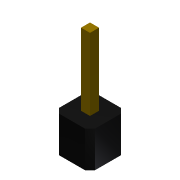
# Autodesk Inventor part: Header1x1
Saved by Autodesk Inventor 2013 (Build 170138000, 138)
## iProperties
Created: 2013-01-19
Part Number: Header1x1
Material: Generic
Document SubType Name: Modeling
Designer: davidgitz
Density: 1 g/cm^3
Author: davidgitz
Autodesk Inventor part; units mm, degrees
ref_plane "YZ Plane" through (0, 0, 0) normal (1, 0, 0) x (0, 1, 0)
ref_plane "XZ Plane" through (0, 0, 0) normal (0, 1, 0) x (-1, 0, 0)
ref_plane "XY Plane" through (0, 0, 0) normal (0, 0, 1) x (1, 0, 0)
sketch "Sketch1" plane through (0, 0, 0) normal (0, 1, 0) x (-1, 0, 0)
  line L0 (0.9108, 1.27) -> (-0.9108, 1.27)
  line L1 (-0.9108, 1.27) -> (-1.27, 0.9108)
  line L2 (-1.27, 0.9108) -> (-1.27, -0.9108)
  line L3 (0.9108, -1.27) -> (1.27, -0.9108)
  line L4 (1.27, -0.9108) -> (1.27, 0.9108)
  line L5 (0.9108, 1.27) -> (1.27, 0.9108)
  line L6 (-1.27, -0.9108) -> (-0.9108, -1.27)
  line L7 (-0.9108, -1.27) -> (0.9108, -1.27)
  line L8 (-1.27, 0) -> (1.27, 0) construction
  point P0 (0, 0)
  point P1 (0, 0)
  dimension "d1" = 2.54
  dimension "d3" = 0.508
  dimension "d4" = 135
  constraints: 18 end point, 10 perpendicular, 3 midpoint, 1 coincident, 1 vertical
  measures "d1" distance between parallel lines of L4 L2
  measures "d3" distance of L0.end L1.end
  measures "d4" angle of L0 L1
extrude "Extrusion1" add sketch "Sketch1" along normal blind 2.54
sketch "Sketch2" plane through (0, 2.54, 0) normal (0, 1, 0) x (1, 0, 0)
  line L0 (-0.3175, 0.3175) -> (0.3175, 0.3175)
  line L1 (0.3175, 0.3175) -> (0.3175, -0.3175)
  line L2 (0.3175, -0.3175) -> (-0.3175, -0.3175)
  line L3 (-0.3175, -0.3175) -> (-0.3175, 0.3175)
  line L4 (-0.3175, 0.3175) -> (0.3175, -0.3175) construction
  point P0 (0, 0)
  point P1 (0, 0)
  dimension "d7" = 0.635
  constraints: 10 end point, 2 parallel, 2 perpendicular, 1 coincident, 1 horizontal, 1 midpoint
  measures "d7" distance of L0.start L0.end
extrude "Extrusion2" add sketch "Sketch2" along normal blind 5.08
body "Solid1"
